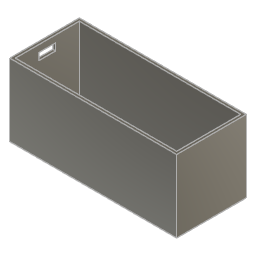
case (Autodesk Fusion 360 design; units mm, degrees)
Autodesk Fusion 360 part; units mm, degrees
sketch "Sketch1" plane through (0, 0, 0) normal (0, 0, 1) x (1, 0, 0)
  line L0 (0, 0) -> (120, 0)
  line L1 (120, 0) -> (120, 50)
  line L2 (120, 50) -> (0, 50)
  line L3 (0, 50) -> (0, 0)
  line L4 (16.75, 41.3333) -> (103.25, 41.3333)
  line L5 (103.25, 41.3333) -> (103.25, 29.3333)
  line L6 (103.25, 29.3333) -> (16.75, 29.3333)
  line L7 (16.75, 29.3333) -> (16.75, 41.3333)
  line L8 (16.75, 20.6667) -> (103.25, 20.6667)
  line L9 (103.25, 20.6667) -> (103.25, 8.6667)
  line L10 (103.25, 8.6667) -> (16.75, 8.6667)
  line L11 (16.75, 8.6667) -> (16.75, 20.6667)
  line L12 (103.25, 35.3656) -> (120, 35.3656) construction
  line L13 (0, 36) -> (16.75, 36) construction
  line L14 (16.75, 14.6667) -> (0, 14.6667) construction
  line L15 (103.25, 14.6667) -> (120, 14.6667) construction
  line L16 (54.6731, 50) -> (54.6731, 41.3333) construction
  line L17 (54.6731, 29.3333) -> (54.6731, 20.6667) construction
  line L18 (56.6135, 8.6667) -> (56.6135, 0) construction
  dimension "d1" = 120
  dimension "d2" = 50
  dimension "d3" = 86.5
  dimension "d4" = 12
  dimension "d6" = 86.5
  dimension "d7" = 12
  constraint horizontal L0
  constraint vertical L1
  constraint horizontal L2
  constraint vertical L3
  constraint coincident L0.start L3.end
  constraint horizontal L4
  constraint vertical L5
  constraint horizontal L6
  constraint vertical L7
  constraint horizontal L8
  constraint vertical L9
  constraint horizontal L10
  constraint vertical L11
  constraint coincident L5 L12.start
  constraint coincident L1 L12.end
  constraint perpendicular L1 L12
  constraint coincident L3 L13.start
  constraint coincident L7 L13.end
  constraint perpendicular L7 L13
  constraint equal L12 L13
  constraint midpoint L11 L14.start
  constraint coincident L3 L14.end
  constraint perpendicular L3 L14
  constraint midpoint L9 L15.start
  constraint coincident L1 L15.end
  constraint perpendicular L1 L15
  constraint equal L14 L15
  constraint coincident L2 L16.start
  constraint coincident L4 L16.end
  constraint perpendicular L4 L16
  constraint coincident L6 L17.start
  constraint coincident L8 L17.end
  constraint perpendicular L8 L17
  constraint coincident L10 L18.start
  constraint coincident L0 L18.end
  constraint perpendicular L0 L18
  constraint equal L16 L18
  constraint equal L16 L17
  measures "d1" distance of L0.start L0.end
  measures "d2" distance of L0.start L2.end
  measures "d3" distance of L4.start L4.end
  measures "d4" distance of L4.start L6.end
  measures "d6" distance of L8.start L8.end
  measures "d7" distance of L8.start L10.end
extrude "Extrude1" add sketch "Sketch1" along normal blind 2
sketch "Sketch2" plane through (0, 0, 2) normal (0, 0, 1) x (-1, 0, 0)
  line L0 (-103.25, -8.6667) -> (-16.75, -8.6667)
  line L1 (-16.75, -8.6667) -> (-16.75, -20.6667)
  line L2 (-16.75, -20.6667) -> (-103.25, -20.6667)
  line L3 (-103.25, -20.6667) -> (-103.25, -8.6667)
  line L4 (-103.25, -29.3333) -> (-16.75, -29.3333)
  line L5 (-16.75, -29.3333) -> (-16.75, -41.3333)
  line L6 (-16.75, -41.3333) -> (-103.25, -41.3333)
  line L7 (-103.25, -41.3333) -> (-103.25, -29.3333)
  line L8 (0, -50) -> (0, 0)
  line L9 (0, 0) -> (-120, 0)
  line L10 (-120, 0) -> (-120, -50)
  line L11 (-120, -50) -> (0, -50)
  line L12 (-2, -48) -> (-118, -48)
  line L13 (-118, -48) -> (-118, -2)
  line L14 (-118, -2) -> (-2, -2)
  line L15 (-2, -2) -> (-2, -48)
  dimension "d10" = 2
  dimension "d11" = 2
  dimension "d12" = 2
  dimension "d13" = 2
  constraint horizontal L12
  constraint vertical L13
  constraint horizontal L14
  constraint vertical L15
  measures "d10" distance of L10 L13
  measures "d11" distance of L8 L15
  measures "d12" distance of L11 L12
  measures "d13" distance of L9 L14
extrude "Extrude2" add sketch "Sketch2" along normal blind 50 contours L8 L9 L10 L11
sketch "Sketch3" plane through (0, 0, 0) normal (-1, 0, 0) x (0, -1, 0)
  line L0 (-50, 0) -> (0, 0)
  line L1 (0, 0) -> (0, 52)
  line L2 (0, 52) -> (-50, 52)
  line L3 (-50, 52) -> (-50, 0)
  line L4 (-31, 47) -> (-19, 47)
  line L5 (-19, 47) -> (-19, 42)
  line L6 (-19, 42) -> (-31, 42)
  line L7 (-31, 42) -> (-31, 47)
  line L8 (-31, 44.5) -> (-50, 44.5) construction
  line L9 (-40.8681, 44.5) -> (-40.5, 44.5) construction
  line L10 (-19, 44.5) -> (0, 44.5) construction
  dimension "d16" = 12
  dimension "d17" = 5
  dimension "d18" = 5
  constraint horizontal L4
  constraint vertical L5
  constraint horizontal L6
  constraint vertical L7
  constraint midpoint L7 L8.start
  constraint coincident L3 L8.end
  constraint perpendicular L3 L8
  constraint coincident L8 L9.start
  constraint midpoint L8 L9.end
  constraint perpendicular L5 L9
  constraint midpoint L5 L10.start
  constraint coincident L1 L10.end
  constraint perpendicular L1 L10
  constraint equal L8 L10
  measures "d16" distance of L4.start L4.end
  measures "d17" distance of L4.end L5.end
  measures "d18" distance of L2 L4
extrude "Extrude3" cut sketch "Sketch3" against normal blind 10 contours L4 L5 L6 L7
